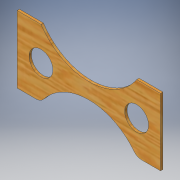
# Autodesk Inventor part: Devant - Haut Rammasse-Balle
Saved by Autodesk Inventor 2016 (Build 200138000, 138)
## iProperties
Created: 2016-01-24
Part Number: Devant - Haut Rammasse-Balle
Material: Generic
Document SubType Name: Modeling
Designer: ares-b02
Density: 1 g/cm^3
Appearance: Plywood - New
Author: ares-b02
Autodesk Inventor part; units mm, degrees
ref_plane "YZ Plane" through (0, 0, 0) normal (1, 0, 0) x (0, 1, 0)
ref_plane "XZ Plane" through (0, 0, 0) normal (0, 1, 0) x (-1, 0, 0)
ref_plane "XY Plane" through (0, 0, 0) normal (0, 0, 1) x (1, 0, 0)
sketch "Sketch1" plane through (0, 0, 0) normal (0, 0, 1) x (1, 0, 0)
  line L0 (167.1611, 130.6481) -> (167.1611, -47.4567)
  line L1 (-213.8389, -47.4567) -> (-213.8389, 130.6481)
  line L2 (-213.8389, -47.4567) -> (-150.3389, -47.4567)
  line L3 (167.1611, -47.4567) -> (103.6611, -47.4567)
  arc A0 (103.6611, -47.4567) -> (-150.3389, -47.4567) centre (-23.3389, -131.699) ccw
  line L4 (-213.8389, 130.6481) -> (-150.3389, 130.6481)
  line L5 (167.1611, 130.6481) -> (103.6611, 130.6481)
  arc A1 (-150.3389, 130.6481) -> (103.6611, 130.6481) centre (-23.3389, 214.8904) ccw
  point P0 (0, 0)
  dimension "d0" = 381
  dimension "d1" = 178.1048
  dimension "d35" = 63.5
  dimension "d36" = 63.5
  dimension "d39" = 152.4
  dimension "d40" = 63.5
  dimension "d41" = 63.5
  dimension "d42" = 152.4
  constraints: 12 end point, 4 horizontal, 4 point on circle, 2 centre point, 1 parallel
  measures "d0" distance of L1.end L0.start
  measures "d1" distance of L1.start L1.end
  measures "d35" distance of L1.start L2.end
  measures "d36" distance of L0.end L3.end
  measures "d39" radius of A0
  measures "d40" distance of L1.end L4.end
  measures "d41" distance of L0.start L5.end
  measures "d42" radius of A1
extrude "Extrusion1" add sketch "Sketch1" along normal blind 6.35
fillet "Fillet1" radius 25.4 2 edges at (-150.3389, -47.4567, 3.175) (103.6611, -47.4567, 3.175)
hole "Hole1" at (-150.3389, 41.5957, 6.35) direction (0, 0, -1) diameter 63.5 end through all
hole "Hole2" at (103.6611, 41.5957, 6.35) direction (0, 0, -1) diameter 63.5 end through all
body "Solid1"
